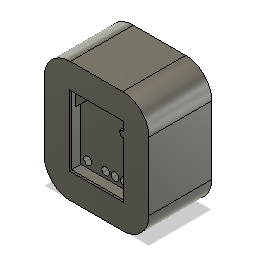
Fomu Hacker Programming Jig v5 (Autodesk Fusion 360 design; units mm, degrees)
Autodesk Fusion 360 part; units mm, degrees
sketch "Sketch1" plane through (0, 0, 0) normal (0, 0, 1) x (1, 0, 0)
  line L0 (0, 0) -> (10, 0)
  line L1 (10, 0) -> (10, 13)
  line L2 (10, 13) -> (0, 13)
  line L3 (0, 13) -> (0, 0)
  line L4 (15, -5) -> (15, 18)
  line L5 (15, 18) -> (-5, 18)
  line L6 (-5, 18) -> (-5, -5)
  line L7 (-5, -5) -> (15, -5)
  dimension "d1" = 10
  dimension "d2" = 13
  dimension "d3" = 5
  measures "d1" distance of L0.start
  measures "d2" distance of L0.start
  measures "d3" distance of L1
extrude "Extrude1" add sketch "Sketch1" along normal blind 7
sketch "Sketch2" plane through (0, 0, 0) normal (0, 0, -1) x (-1, 0, 0)
  line L0 (0, 13) -> (0, 0)
  line L1 (0, 0) -> (-10, 0)
  line L2 (-10, 0) -> (-10, 13)
  line L3 (-10, 13) -> (0, 13)
  line L4 (-15, -5) -> (5, -5)
  line L5 (5, -5) -> (5, 18)
  line L6 (5, 18) -> (-15, 18)
  line L7 (-15, 18) -> (-15, -5)
extrude "Extrude2" add sketch "Sketch2" against normal blind 5 contours L0 L1 L2 L3
sketch "Sketch3" plane through (0, 0, 5) normal (0, 0, 1) x (1, 0, 0)
  line L0 (10, 0) -> (10, 13)
  line L1 (10, 13) -> (0, 13)
  line L2 (0, 13) -> (0, 0)
  line L3 (0, 0) -> (10, 0)
  line L4 (0, 10) -> (3, 13)
  line L5 (0, 13) -> (3, 13)
  line L6 (0, 13) -> (0, 10)
  dimension "d73" = 3
  dimension "d74" = 3
extrude "Extrude3" add sketch "Sketch3" along normal blind 1 contours L1 L2 L4 L5 L6
sketch "Sketch4" plane through (0, 0, 5) normal (0, 0, 1) x (1, 0, 0)
  line L0 (10, 13) -> (3, 13)
  line L1 (0, 10) -> (0, 0)
  line L2 (0, 0) -> (10, 0)
  line L3 (10, 0) -> (10, 13)
  circle A0 centre (1.3, 1.25) radius 0.75
  circle A1 centre (9, 8.2) radius 0.75
  circle A2 centre (9, 5.3) radius 0.75
  circle A3 centre (9, 3.3) radius 0.75
  circle A4 centre (8.35, 1.25) radius 0.75
  circle A5 centre (6.5, 1.25) radius 0.75
  circle A6 centre (4.75, 1.25) radius 0.75
  line L4 (3, 13) -> (0, 10)
  dimension "d12" = 3.3
  dimension "d14" = 5.3
  dimension "d15" = 8.2
  dimension "d16" = 1.5
  dimension "d17" = 1.5
  dimension "d18" = 1.5
  dimension "d19" = 1.25
  dimension "d21" = 1.5
  dimension "d22" = 1.5
  dimension "d23" = 1.5
  dimension "d24" = 1.5
  dimension "d68" = 1
  dimension "d69" = 1.65
  dimension "d70" = 3.5
  dimension "d71" = 5.25
  dimension "d72" = 8.7
  measures "d12" distance of L1.end
  measures "d14" distance of L1.end
  measures "d15" distance of L1.end
  measures "d16" diameter of A3
  measures "d17" diameter of A2
  measures "d18" diameter of A1
  measures "d19" distance of L1.end
  measures "d21" diameter of A4
  measures "d22" diameter of A5
  measures "d23" diameter of A6
  measures "d24" diameter of A0
extrude "Extrude4" cut sketch "Sketch4" against normal blind 8.5 contours A0 | A1 | A2 | A3 | A4 | A5 | A6
sketch "Sketch5" plane through (0, 0, 0) normal (0, 0, -1) x (-1, 0, 0)
  circle A0 centre (-6.5, 1.25) radius 0.75
  circle A1 centre (-9, 8.2) radius 0.75
  circle A2 centre (-8.35, 1.25) radius 0.75
  circle A3 centre (-4.75, 1.25) radius 0.75
  circle A4 centre (-9, 5.3) radius 0.75
  circle A5 centre (-9, 3.3) radius 0.75
  circle A6 centre (-1.3, 1.25) radius 0.75
  line L0 (-15, -5) -> (5, -5)
  line L1 (5, -5) -> (5, 18)
  line L2 (5, 18) -> (-15, 18)
  line L3 (-15, 18) -> (-15, -5)
  line L4 (-2.2, 2.15) -> (-0.4, 2.15)
  line L5 (-0.4, 2.15) -> (-0.4, 0.35)
  line L6 (-0.4, 0.35) -> (-2.2, 0.35)
  line L7 (-2.2, 0.35) -> (-2.2, 2.15)
  line L8 (-5.65, 2.15) -> (-3.85, 2.15)
  line L9 (-3.85, 2.15) -> (-3.85, 0.35)
  line L10 (-3.85, 0.35) -> (-5.65, 0.35)
  line L11 (-5.65, 0.35) -> (-5.65, 2.15)
  line L12 (-7.4, 2.15) -> (-5.6, 2.15)
  line L13 (-5.6, 2.15) -> (-5.6, 0.35)
  line L14 (-5.6, 0.35) -> (-7.4, 0.35)
  line L15 (-7.4, 0.35) -> (-7.4, 2.15)
  line L16 (-9.25, 2.15) -> (-7.45, 2.15)
  line L17 (-7.45, 2.15) -> (-7.45, 0.35)
  line L18 (-7.45, 0.35) -> (-9.25, 0.35)
  line L19 (-9.25, 0.35) -> (-9.25, 2.15)
  line L20 (-9.9, 4.2) -> (-8.1, 4.2)
  line L21 (-8.1, 4.2) -> (-8.1, 2.4)
  line L22 (-8.1, 2.4) -> (-9.9, 2.4)
  line L23 (-9.9, 2.4) -> (-9.9, 4.2)
  line L24 (-9.9, 6.2) -> (-8.1, 6.2)
  line L25 (-8.1, 6.2) -> (-8.1, 4.4)
  line L26 (-8.1, 4.4) -> (-9.9, 4.4)
  line L27 (-9.9, 4.4) -> (-9.9, 6.2)
  line L28 (-9.9, 9.1) -> (-8.1, 9.1)
  line L29 (-8.1, 9.1) -> (-8.1, 7.3)
  line L30 (-8.1, 7.3) -> (-9.9, 7.3)
  line L31 (-9.9, 7.3) -> (-9.9, 9.1)
  dimension "d31" = 1.8
  dimension "d32" = 1.8
  dimension "d33" = 1.8
  dimension "d34" = 1.8
  dimension "d35" = 1.8
  dimension "d36" = 1.8
  dimension "d37" = 1.8
  dimension "d38" = 1.8
  dimension "d39" = 1.8
  dimension "d40" = 1.8
  dimension "d41" = 1.8
  dimension "d42" = 1.8
  dimension "d43" = 1.8
  dimension "d44" = 1.8
  dimension "d45" = 0.9
  dimension "d46" = 0.9
  dimension "d47" = 0.9
  dimension "d48" = 0.9
  dimension "d49" = 0.9
  dimension "d50" = 0.9
  dimension "d51" = 0.9
  dimension "d52" = 0.9
  dimension "d53" = 0.9
  dimension "d54" = 0.9
  dimension "d55" = 0.9
  dimension "d56" = 0.9
  dimension "d57" = 0.9
  dimension "d58" = 0.9
  measures "d47" distance of L11
  measures "d48" distance of L8
  measures "d49" distance of L12
  measures "d50" distance of L15
  measures "d51" distance of L19
  measures "d52" distance of L18
  measures "d53" distance of L20
  measures "d54" distance of L21
  measures "d55" distance of L25
  measures "d56" distance of L24
  measures "d57" distance of L28
  measures "d58" distance of L31
extrude "Extrude5" add sketch "Sketch5" along normal blind 5 contours L0 L1 L2 L3
fillet "Fillet2" radius 5 4 edges at (15, 18, 1) (-5, 18, 1) (15, -5, 1) (-5, -5, 1)
chamfer "Chamfer1" distance 0.5 angle 45 20 edges at (9, 9.1, -5) (9.9, 8.2, -5) (8.1, 8.2, -5) (9, 7.3, -5) (9, 6.2, -5) (9.9, 5.3, -5) (8.1, 5.3, -5) (8.1, 3.3, -5) (9, 2.4, -5) (9.9, 3.3, -5) (8.35, 2.15, -5) (9.25, 1.25, -5) (8.35, 0.35, -5) (5.625, 2.15, -5) (5.625, 0.35, -5) (3.85, 1.25, -5) (2.2, 1.25, -5) (1.3, 2.15, -5) (0.4, 1.25, -5) (1.3, 0.35, -5)
sketch "Sketch6" plane through (0, 0, 7) normal (0, 0, 1) x (1, 0, 0)
  arc A0 (-5, 0) -> (0, -5) centre (0, 0) ccw
  line L0 (0, -5) -> (10, -5)
  arc A1 (10, -5) -> (15, 0) centre (10, 0) ccw
  line L1 (15, 0) -> (15, 13)
  arc A2 (15, 13) -> (10, 18) centre (10, 13) ccw
  line L2 (10, 18) -> (0, 18)
  arc A3 (0, 18) -> (-5, 13) centre (0, 13) ccw
  line L3 (-5, 13) -> (-5, 0)
  line L4 (0, 0) -> (0, 13)
  line L5 (0, 13) -> (10, 13)
  line L6 (10, 13) -> (10, 0)
  line L7 (10, 0) -> (0, 0)
  arc A4 (10, 11.75) -> (10, 10.25) centre (10, 11) ccw
  line L8 (10, 11.75) -> (10, 10.25)
  dimension "d63" = 1.5
  dimension "d64" = 11
  measures "d63" diameter of A4
extrude "Extrude6" add sketch "Sketch6" against normal blind 2 contours L6 A4 L8
chamfer "Chamfer2" distance 0.2 angle 45 6 edges at (5, 13, 7) (10, 12.375, 7) (9.25, 11, 7) (10, 5.125, 7) (5, 0, 7) (0, 6.5, 7)
equation "d16 = d18"
equation "d17 = d18"
equation "d21 = d18"
equation "d22 = d18"
equation "d23 = d18"
equation "d24 = d18"
equation "d31 = d44"
equation "d32 = d44"
equation "d33 = d44"
equation "d34 = d40"
equation "d35 = d40"
equation "d36 = d40"
equation "d37 = d39"
equation "d38 = d40"
equation "d39 = d44"
equation "d40 = d44"
equation "d41 = d44"
equation "d42 = d44"
equation "d43 = d44"
equation "d45 = d43 / 2"
equation "d46 = d44 / 2"
equation "d47 = d41 / 2"
equation "d48 = d42 / 2"
equation "d49 = d40 / 2"
equation "d50 = d39 / 2"
equation "d51 = d37 / 2"
equation "d52 = d38 / 2"
equation "d53 = d36 / 2"
equation "d54 = d35 / 2"
equation "d55 = d33 / 2"
equation "d56 = d34 / 2"
equation "d57 = d32 / 2"
equation "d58 = d31 / 2"
